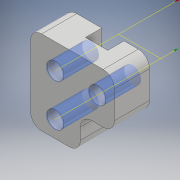
# Autodesk Inventor part: piano_wire_back_fixation
Saved by Autodesk Inventor 2018 (Build 220112000, 112)
## iProperties
Created: 2018-04-24
Part Number: piano_wire_back_fixation
Material: Generic
Document SubType Name: Modeling
Designer: medrimonia
Density: 1 g/cm^3
Appearance: Default
Vendor: Rhoban
Mass: 0.876766 g
Surface Area: 8.68852 cm^2
Volume: 0.876766 cm^3
side_2_corner: 7,500 mm
wire_diameter: 3,000 mm
wire_2_corner: 2,000 mm
Author: medrimonia
Autodesk Inventor part; units mm, degrees
ref_plane "YZ Plane" through (0, 0, 0) normal (1, 0, 0) x (0, 1, 0)
ref_plane "XZ Plane" through (0, 0, 0) normal (0, 1, 0) x (-1, 0, 0)
ref_plane "XY Plane" through (0, 0, 0) normal (0, 0, 1) x (1, 0, 0)
sketch "Sketch1" plane through (0, 0, 0) normal (0, 1, 0) x (-1, 0, 0)
  line L0 (0, 0) -> (7.5, 0) construction
  line L1 (7.5, 0) -> (7.5, -7.5) construction
  line L2 (0, 0) -> (-3, 0) construction
  line L3 (-3, -4.45) -> (-3, 4.45)
  line L4 (-3, 4.45) -> (11.95, 4.45)
  line L5 (11.95, 4.45) -> (11.95, -10.5)
  line L6 (11.95, -10.5) -> (3.05, -10.5)
  line L7 (3.05, -10.5) -> (3.05, -4.45)
  line L8 (3.05, -4.45) -> (-3, -4.45)
  line L9 (7.5, -7.5) -> (7.5, -10.5) construction
  dimension "d0" = 7.5
  dimension "d1" = 7.5
  dimension "d2" = 8.9
  dimension "d3" = 3
  constraints: 20 end point, 6 perpendicular, 3 coincident, 3 horizontal, 3 vertical, 2 midpoint
  measures "d0" distance of L0.start L0.end
  measures "d1" distance of L0.end L1.end
  measures "d2" distance of L3.start L3.end
  measures "d3" distance of L2.start L2.end
extrude "Extrusion1" add sketch "Sketch1" along normal blind 6.25
hole "Hole1" at (0, 0, 0) at (-7.5, 0, 0) at (-7.5, 0, -7.5) direction (0, 1, 0) diameter 3 end through all
sketch "Sketch2" plane through (0, 6.25, 0) normal (0, 1, 0) x (1, 0, 0)
  circle A0 centre (-7.5, 0) radius 1.5 projected
  circle A1 centre (0, 0) radius 1.5 construction
  circle A2 centre (-7.5, 7.5) radius 1.5 projected
  line L0 (3, -4.45) -> (3, 4.45) construction
  line L1 (3, 4.45) -> (-3.05, 4.45) construction
  line L2 (-3.05, 4.45) -> (-3.05, 10.5) construction
  line L3 (-3.05, 10.5) -> (-11.95, 10.5) construction
  line L4 (-11.95, 10.5) -> (-11.95, -4.45) construction
  line L5 (-11.95, -4.45) -> (3, -4.45) construction
  line L6 (-11.95, -4.45) -> (-11.95, 10.5) projected
  line L7 (-11.95, 2) -> (-7, 2)
  line L8 (-5.5, 2) -> (-5.5, 0.5) construction
  line L9 (-11.95, -4.45) -> (3, -4.45) construction
  line L10 (-3.05, 4.45) -> (3, 4.45) construction
  line L11 (-7.5, 0) -> (-7.5, 2) construction
  line L12 (-7.5, 0) -> (-5.5, 0) construction
  line L13 (-3.05, 4.45) -> (-3.05, 10.5) construction
  line L14 (-3.05, 10.5) -> (-3.05, 4.45) construction
  line L15 (-1.5378, -4.45) -> (-5.5, -4.45)
  line L16 (-11.95, 2) -> (-11.95, 5.9622)
  line L17 (-11.95, 10.5) -> (-11.95, -4.45) projected
  line L18 (-11.95, 5.9622) -> (-6.5633, 5.4909)
  line L19 (-1.5378, -4.45) -> (-2.0091, 0.9367)
  circle A3 centre (-7, 0.5) radius 1.5
  line L20 (-7, 2) -> (-5.5, 2) construction
  line L21 (-5.5, 0.5) -> (-5.5, -4.45)
  arc A4 (-2.0091, 0.9367) -> (-6.5633, 5.4909) centre (-7, 0.5) ccw
  dimension "d14" = 2
  dimension "d18" = 5
  dimension "d19" = 5
  dimension "d21" = 3
  dimension "d22" = 5.01
  constraints: 23 end point, 13 perpendicular, 8 point on line, 6 tangent, 4 point on circle, 2 centre point, 2 collinear, 1 coincident
  measures "d14" distance of L11.start L11.end
  measures "d18" angle of L8 L19
  measures "d19" angle of L7 L18
  measures "d21" diameter of A3
  measures "d22" radius of A4
extrude "MontageEnForce" cut sketch "Sketch2" against normal blind 2.9 contours L7 L6 L18 A4 L19 L15 L21 A3
fillet "Fillet1" radius 2 6 edges at (-3.05, 3.125, -4.45) (-11.95, 3.125, 4.45) (-3.05, 3.125, -10.5) (-11.95, 3.125, -10.5) (3, 3.125, 4.45) (3, 3.125, -4.45)
ref_plane "Work Plane1" through (0, 4.8, 0) normal (0, 1, 0) x (1, 0, 0)
sketch "Sketch4" plane through (0, 6.25, 0) normal (0, 1, 0) x (1, 0, 0)
  circle A0 centre (-7.5, 0) radius 1.5 projected
  circle A1 centre (-7.5, 7.5) radius 1.5 projected
  circle A2 centre (0, 0) radius 1.5 projected
ref_plane "Work Plane5" through (-7.5, 6.25, 0) normal (-1, 0, 0) x (0, 0, 1)
ref_plane "Work Plane6" through (0, 6.25, 0) normal (-1, 0, 0) x (0, 0, 1)
ref_plane "Work Plane7" through (-7.5, 6.25, 0) normal (0, 0, 1) x (1, 0, 0)
ref_plane "Work Plane8" through (-7.5, 6.25, -7.5) normal (0, 0, 1) x (1, 0, 0)
ref_plane "Work Plane2" through (-3.75, 6.25, 0) normal (-1, 0, 0) x (0, 0, 1)
ref_plane "Work Plane3" through (-7.5, 6.25, -3.75) normal (0, 0, 1) x (1, 0, 0)
equation "\"d0\" = side_2_corner"
equation "\"d1\" = side_2_corner"
equation "\"d2\" = width"
equation "\"d3\" = hole_2_border"
equation "\"d4\" = fix_thickness"
equation "\"d14\" = wire_2_corner"
equation "\"d18\" = angle_tol"
equation "\"d19\" = angle_tol"
equation "\"d21\" = 2 * wire_corner_fillet"
equation "\"d22\" = wire_corner_margin + wire_diameter + wire_corner_fillet"
equation "\"fix_thickness\" = 6.25"
equation "\"wire_diameter\" = 3"
equation "\"back_fix_width\" = 1"
equation "\"side_2_corner\" = piano_wire_holes_spacing"
equation "\"wire_2_corner\" = 2"
equation "\"angle_tol\" = 5deg"
equation "\"wire_corner_margin\" = 0.51"
equation "\"wire_corner_fillet\" = 1.5"
equation "\"hole_2_border\" = 3"
equation "\"width\" = 8.9"
equation "\"piano_wire_holes_spacing\" = 7.5"
body "Solid1"
